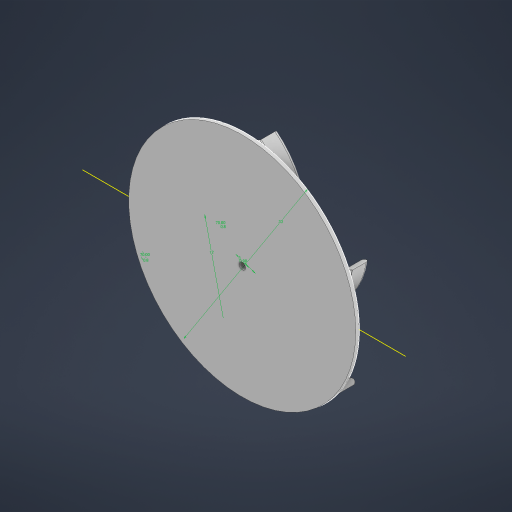
# Autodesk Inventor part: fan-concreate
Saved by Autodesk Inventor 2023.5 (Build 275446000, 446)
## iProperties
Created: 2025-01-28
Part Number: fan-concreate
Material: 一般
Document SubType Name: Modeling
Designer: IshiiLabHonda
Density: 1 g/cm^3
Appearance: 既定
Author: IshiiLabHonda
Autodesk Inventor part; units mm, degrees
ref_plane "YZ Plane" through (0, 0, 0) normal (1, 0, 0) x (0, 1, 0)
ref_plane "XZ Plane" through (0, 0, 0) normal (0, 1, 0) x (-1, 0, 0)
ref_plane "XY Plane" through (0, 0, 0) normal (0, 0, 1) x (1, 0, 0)
sketch "スケッチ1" plane through (0, 0, 0) normal (0, 0, 1) x (1, 0, 0)
  circle A0 centre (0, 0) radius 16.5
  circle A1 centre (0, 0) radius 0.49
  dimension "d0" = 33
  dimension "d1" = 0.98
  constraints: 2 centre point, 2 coincident
  measures "d0" diameter of A0
  measures "d1" diameter of A1
extrude "押し出し1" add sketch "スケッチ1" along normal blind 0.5
sketch "スケッチ2" plane through (0, 0, 0) normal (0, 0, 1) x (1, 0, 0)
  circle A0 centre (0, 0) radius 1.5
  circle A1 centre (0, 0) radius 16.5 projected
  circle A2 centre (0, 0) radius 0.49 projected
  arc A3 (-3.2671, 3.5664) -> (-15.1253, -6.5937) centre (-3.2671, -8.4336) ccw
  line L0 (-23.7047, 0) -> (23.2008, 0) projected
  line L1 (-3.2671, 3.5664) -> (-3.5408, 2.8147)
  line L2 (-15.1253, -6.5937) -> (-14.3404, -6.4386)
  arc A4 (-3.5408, 2.8147) -> (-14.3404, -6.4386) centre (-2.6513, -9.1523) ccw
  line L3 (-15.1253, -6.5937) -> (-14.7476, -4.16) construction
  line L4 (-3.2671, 3.5664) -> (-3.7005, 3.5664) construction
  dimension "d4" = 3
  dimension "d6" = 12
  dimension "d9" = 70
  dimension "d10" = 70
  dimension "d11" = 0.8
  dimension "d12" = 0.8
  constraints: 8 end point, 7 point on circle, 3 centre point, 2 tangent, 1 coincident, 1 parallel
  measures "d4" diameter of A0
  measures "d6" radius of A3
  measures "d9" angle of L2 L3
  measures "d10" angle of L1 L4
  measures "d11" distance of L1.start L1.end
  measures "d12" distance of L2.start L2.end
extrude "押し出し3" add sketch "スケッチ2" against normal blind 4 contours L0 A2 A0 | A0 L0 A2
fillet "フィレット1" radius 2 1 edges at (-1.5, 0, 0)
fillet "フィレット2" radius 0.4 1 edges at (-1.5, 0, -4)
extrude "押し出し2" add sketch "スケッチ2" against normal blind 2.8 contours A4 L2 A3 L0 | L0 A3 L1 A4
fillet "フィレット3" radius 0.4 3 edges at (-11.0749, 0.679, -2.8) (-10.4591, -0.0397, -2.8) (-14.7328, -6.5161, 0)
fillet "フィレット4" radius 0.4 2 edges at (-10.623, -0.1828, 0) (-11.0749, 0.679, 0)
pattern_circular "円形状パターン2" count 6 over 360 about axis through (0, 0, -10) along (0, 0, 1) of "押し出し2", "フィレット3", "フィレット4"
